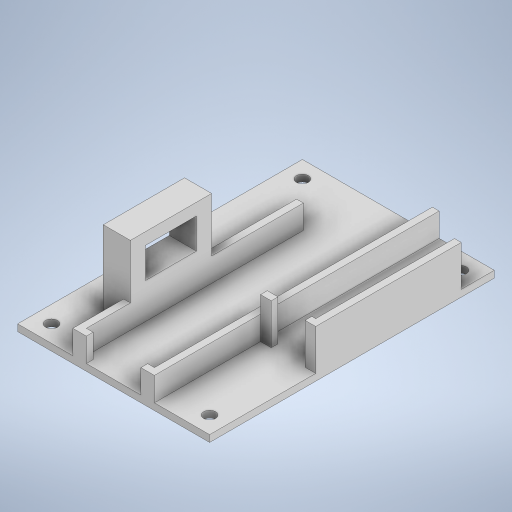
# Autodesk Inventor part: light_indicator
Saved by Autodesk Inventor 2023 (Build 270158000, 158)
## iProperties
Created: 2024-04-16
Part Number: light_indicator
Material: Genérico
Document SubType Name: Modeling
Designer: inigo
Density: 1 g/cm^3
Appearance: Valor por defecto
Author: inigo
Autodesk Inventor part; units mm, degrees
ref_plane "YZ Plane" through (0, 0, 0) normal (1, 0, 0) x (0, 1, 0)
ref_plane "XZ Plane" through (0, 0, 0) normal (0, 1, 0) x (-1, 0, 0)
ref_plane "XY Plane" through (0, 0, 0) normal (0, 0, 1) x (1, 0, 0)
sketch "Boceto1" plane through (0, 0, 0) normal (0, 1, 0) x (-1, 0, 0)
  line L0 (10.05, 40.05) -> (-10.05, 40.05)
  line L1 (-10.05, 40.05) -> (-10.05, -40.05)
  line L2 (-10.05, -40.05) -> (10.05, -40.05)
  line L3 (10.05, -40.05) -> (10.05, 40.05)
  line L4 (10.05, 40.05) -> (-10.05, -40.05) construction
  line L5 (-10.05, 40.05) -> (10.05, -40.05) construction
  line L6 (12.05, 42.05) -> (-12.05, 42.05)
  line L7 (-12.05, 42.05) -> (-12.05, -42.05)
  line L8 (-12.05, -42.05) -> (12.05, -42.05)
  line L9 (12.05, -42.05) -> (12.05, 42.05)
  point P0 (0, 0)
  dimension "d0" = 20.1
  dimension "d1" = 80.1
  dimension "d2" = 2
  constraints: 20 end point, 4 parallel, 2 midpoint, 2 perpendicular, 1 horizontal, 3 other
  measures "d0" distance of L2.end L1.end
  measures "d1" distance of L1.end L0.end
  measures "d2" distance between parallel lines of L3 L9
extrude "Extrusión1" add sketch "Boceto1" along normal blind 2 contours L3 L2 L1 L0 | L9 L8 L7 L6
sketch "Boceto2" plane through (0, 2, 0) normal (0, 1, 0) x (1, 0, 0)
  line L0 (12.05, -42.05) -> (12.05, 42.05) projected
  line L1 (-12.05, -42.05) -> (12.05, -42.05)
  line L2 (12.05, -42.05) -> (12.05, 42.05)
  line L3 (-12.05, 42.05) -> (-12.05, -42.05)
  line L4 (-12.05, -42.05) -> (12.05, 42.05) construction
  line L5 (12.05, -42.05) -> (-12.05, 42.05) construction
  line L6 (-10.05, -40.05) -> (10.05, -40.05)
  line L7 (10.05, -40.05) -> (10.05, 40.15)
  line L8 (-10.05, 40.05) -> (-10.05, -40.05)
  line L9 (-10.05, 40.05) -> (-10.05, 42.05)
  line L10 (10.05, 40.15) -> (10.05, 42.05)
  line L11 (12.05, 42.05) -> (-12.05, 42.05) projected
  line L12 (12.05, 42.05) -> (10.05, 42.05)
  line L13 (-12.05, 42.05) -> (-10.05, 42.05)
  line L14 (-12.05, 42.05) -> (-12.05, -42.05) projected
  line L15 (-12.05, 24.05) -> (-10.05, 24.05)
  line L16 (-12.05, -27.6873) -> (-10.05, -27.6873)
  line L17 (-10.05, -27.6873) -> (-10.05, -12.6873)
  line L18 (-10.05, -12.6873) -> (-12.05, -12.6873)
  line L19 (-12.05, -12.6873) -> (-12.05, -27.6873)
  line L20 (-8.05, -40.05) -> (-8.05, -42.05)
  line L21 (-12.05, -42.05) -> (12.05, -42.05) projected
  line L22 (8.05, -40.05) -> (8.05, -42.05)
  point P0 (0, 0)
  point P1 (8.05, -41.05)
  point P2 (-12.05, 24.05)
  dimension "d5" = 2
  dimension "d8" = 18
  dimension "d9" = 15
  dimension "d10" = 12.3627
  dimension "d11" = 2
  dimension "d12" = 2
  dimension "d13" = 4
  dimension "d14" = 4
  constraints: 38 end point, 8 point on line, 6 perpendicular, 4 parallel, 3 midpoint, 2 horizontal, 1 collinear, 1 vertical, 1 other
  measures "d5" distance between parallel lines of L3 L8
  measures "d8" distance between parallel lines of L11 L15
  measures "d9" distance of L17.end L16.end
  measures "d10" distance between parallel lines of L6 L16
  measures "d11" distance between parallel lines of L1 L6
  measures "d12" distance between parallel lines of L0 L7
  measures "d13" distance between parallel lines of L3 L20
  measures "d14" distance from line of L2 point (8.05, -41.05)
extrude "Extrusión2" add sketch "Boceto2" along normal blind 7 contours L1 L22 L6 L7 L10 L11 L0 | L1 L3 L16 L8 L6 L20 | L3 L18 L8 L16 | L8 L18 L3 L15
sketch "Boceto5" plane through (0, 0, 0) normal (0, 1, 0) x (-1, 0, 0)
  line L0 (-12.05, -30.296) -> (-26.35, -30.296)
  line L1 (-26.35, -30.296) -> (-26.35, 8.704)
  line L2 (-26.35, 8.704) -> (-12.05, 8.704)
  line L3 (-12.05, 8.704) -> (-12.05, -30.296)
  line L4 (-12.05, -30.296) -> (-26.35, 8.704) construction
  line L5 (-26.35, -30.296) -> (-12.05, 8.704) construction
  line L6 (-12.05, 42.05) -> (-12.05, -42.05) projected
  line L7 (-28.35, -32.296) -> (-10.05, -32.296)
  line L8 (-10.05, -32.296) -> (-10.05, 10.704)
  line L9 (-10.05, 10.704) -> (-28.35, 10.704)
  line L10 (-28.35, 10.704) -> (-28.35, -32.296)
  point P0 (0, 0)
  point P1 (-19.2, -10.796)
  point P2 (-12.05, 10.704)
  point P3 (-12.05, -32.296)
  dimension "d25" = 14.3
  dimension "d26" = 39
  dimension "d27" = 0
  dimension "d28" = 2
  constraints: 20 end point, 4 parallel, 2 midpoint, 2 perpendicular, 1 horizontal, 3 other
  measures "d25" distance of L1.end L2.end
  measures "d26" distance between parallel lines of L2 L0
  measures "d27" distance between parallel lines of L6 L3
  measures "d28" distance between parallel lines of L0 L7
extrude "Extrusión5" add sketch "Boceto5" along normal blind 14 contours L6 L7 L10 L9 L2 L1 L0 | L0 L1 L2 L3
sketch "Boceto6" plane through (0, 14, 0) normal (0, 1, 0) x (1, 0, 0)
  line L0 (28.35, 32.296) -> (12.05, 32.296) projected
  line L1 (20.2, 32.296) -> (20.2, 4.5557)
  line L2 (14.05, 30.296) -> (26.35, 30.296)
  line L3 (26.35, 30.296) -> (26.35, -8.704)
  line L4 (26.35, -8.704) -> (14.05, -8.704)
  line L5 (14.05, 30.296) -> (26.35, -8.704) construction
  line L6 (26.35, 30.296) -> (14.05, -8.704) construction
  line L7 (28.35, -10.704) -> (28.35, 32.296) projected
  line L8 (12.05, -10.704) -> (28.35, -10.704) projected
  line L9 (14.05, -8.704) -> (12.05, -8.704)
  line L10 (12.05, -8.704) -> (12.05, 30.296)
  line L11 (12.05, 32.296) -> (12.05, -10.704) projected
  line L12 (14.05, 30.296) -> (12.05, 30.296)
  line L13 (28.35, -10.704) -> (28.35, 32.296) projected
  line L14 (28.35, -8.704) -> (28.35, -10.704)
  line L15 (12.05, -10.704) -> (28.35, -10.704) projected
  line L16 (15.2, -8.704) -> (25.2, -8.704)
  line L17 (25.2, -8.704) -> (25.2, -10.704)
  line L18 (25.2, -10.704) -> (15.2, -10.704)
  line L19 (15.2, -10.704) -> (15.2, -8.704)
  line L20 (15.2, -8.704) -> (25.2, -10.704) construction
  line L21 (25.2, -8.704) -> (15.2, -10.704) construction
  line L22 (26.35, 30.296) -> (26.35, 32.296)
  point P0 (0, 0)
  point P1 (20.2, 10.796)
  point P2 (20.2, -8.704)
  point P3 (20.2, -9.704)
  point P4 (15.2, -8.704)
  point P5 (15.2, -10.704)
  point P6 (25.2, -10.704)
  dimension "d31" = 2
  dimension "d32" = 2
  dimension "d33" = 2
  dimension "d34" = 10
  constraints: 34 end point, 6 midpoint, 5 point on line, 4 perpendicular, 3 horizontal, 3 parallel, 1 collinear, 1 vertical
  measures "d31" distance between parallel lines of L7 L3
  measures "d32" distance between parallel lines of L0 L2
  measures "d33" distance from line of L8 point (20.2, -8.704)
  measures "d34" distance of L17.end L18.end
extrude "Extrusión6" cut sketch "Boceto6" against normal blind 12 contours L22 L2 L1 L0 | L1 L2 L12 L11 L0 | L3 L4 L9 L10 L12 L2 | L8 L19 L4 L17
sketch "Boceto8" plane through (0, 0, 0) normal (0, 1, 0) x (-1, 0, 0)
  line L0 (12.05, 27.05) -> (18.05, 27.05)
  line L1 (18.05, 27.05) -> (18.05, 3.05)
  line L2 (18.05, 3.05) -> (12.05, 3.05)
  line L3 (12.05, 3.05) -> (12.05, 27.05)
  line L4 (12.05, -24.05) -> (12.05, 42.05) projected
  line L5 (8.05, 42.05) -> (-8.05, 42.05) projected
  point P0 (0, 0)
  dimension "d44" = 6
  dimension "d45" = 24
  dimension "d46" = 0
  dimension "d47" = 15
  constraints: 8 end point, 2 parallel, 1 horizontal, 1 perpendicular
  measures "d44" distance of L1.end L2.end
  measures "d45" distance of L0.end L1.end
  measures "d46" distance between parallel lines of L4 L3
  measures "d47" distance between parallel lines of L5 L0
extrude "Extrusión8" add sketch "Boceto8" along normal blind 25
sketch "Boceto10" plane through (0, 9, 0) normal (0, 1, 0) x (1, 0, 0)
  line L0 (-12.05, -3.05) -> (-18.05, -3.05) projected
  line L1 (-10.05, -40.05) -> (-10.05, 24.05) projected
  line L2 (-12.05, -3.05) -> (-10.05, -3.05)
  line L3 (-10.05, -3.05) -> (-10.05, -27.05)
  line L4 (-10.05, -27.05) -> (-12.05, -27.05)
  line L5 (-12.05, -27.05) -> (-12.05, -3.05)
  line L6 (-18.05, -27.05) -> (-12.05, -27.05) projected
  point P0 (0, 0)
  point P1 (-10.05, -3.05)
  point P2 (-11.05, -27.05)
  dimension "d65" = 0
  constraints: 8 end point, 2 parallel, 1 horizontal, 1 midpoint, 1 perpendicular, 1 point on line
  measures "d65" distance from line of L6 point (-11.05, -27.05)
extrude "Extrusión10" add sketch "Boceto10" along normal blind 16
sketch "Boceto11" plane through (-18.05, 0, 3.05) normal (-1, 0, 0) x (0, 0, 1)
  line L0 (4.5, 21.5) -> (19.5, 21.5)
  line L1 (19.5, 21.5) -> (19.5, 12.5)
  line L2 (19.5, 12.5) -> (4.5, 12.5)
  line L3 (4.5, 12.5) -> (4.5, 21.5)
  line L4 (4.5, 21.5) -> (19.5, 12.5) construction
  line L5 (19.5, 21.5) -> (4.5, 12.5) construction
  line L6 (0, 25) -> (24, 25) projected
  line L7 (-27.1, 9) -> (0, 9) projected
  line L8 (24, 25) -> (0, 25) projected
  line L9 (12, 25) -> (12, 17)
  point P0 (-3.05, 0)
  dimension "d59" = 15
  dimension "d60" = 9
  dimension "d61" = 3.5
  dimension "d62" = 3.5
  dimension "d66" = 0
  constraints: 14 end point, 4 midpoint, 2 parallel, 2 perpendicular, 1 horizontal
  measures "d59" distance of L1.end L2.end
  measures "d60" distance of L0.end L1.end
  measures "d61" distance between parallel lines of L6 L0
  measures "d62" distance between parallel lines of L7 L2
  measures "d66" distance from line of L9 point (12, 17)
extrude "Extrusión11" cut sketch "Boceto11" against normal blind 8
sketch "Boceto13" plane through (0, 0, 0) normal (0, 1, 0) x (-1, 0, 0)
  line L0 (28.35, -42.05) -> (-28.35, -42.05)
  line L1 (-28.35, -42.05) -> (-28.35, 42.05)
  line L2 (-28.35, 42.05) -> (28.35, 42.05)
  line L3 (28.35, 42.05) -> (28.35, -42.05)
  line L4 (28.35, -42.05) -> (-28.35, 42.05) construction
  line L5 (-28.35, -42.05) -> (28.35, 42.05) construction
  line L6 (-28.35, 10.704) -> (-28.35, -32.296) projected
  line L7 (-8.05, 42.05) -> (-12.05, 42.05) projected
  circle A0 centre (23.35, -37.05) radius 1.75
  line L8 (-12.05, -42.05) -> (12.05, -42.05) projected
  line L9 (0, -42.05) -> (0, -48.6371)
  line L10 (28.35, 0) -> (35.954, 0)
  circle A1 centre (-23.35, -37.05) radius 1.75
  circle A2 centre (23.35, 37.05) radius 1.75
  circle A3 centre (-23.35, 37.05) radius 1.75
  point P0 (0, 0)
  dimension "d67" = 0
  dimension "d68" = 0
  dimension "d72" = 3.5
  dimension "d73" = 5
  dimension "d74" = 5
  constraints: 16 end point, 4 centre point, 4 midpoint, 3 symmetric about line, 2 horizontal, 2 parallel, 1 perpendicular, 1 vertical, 3 other
  measures "d67" distance between parallel lines of L6 L1
  measures "d68" distance between parallel lines of L7 L2
  measures "d72" diameter of A0
  measures "d73" distance from line of L0 A0.centre
  measures "d74" distance from line of L3 A0.centre
extrude "Extrusión12" add sketch "Boceto13" along normal blind 2
